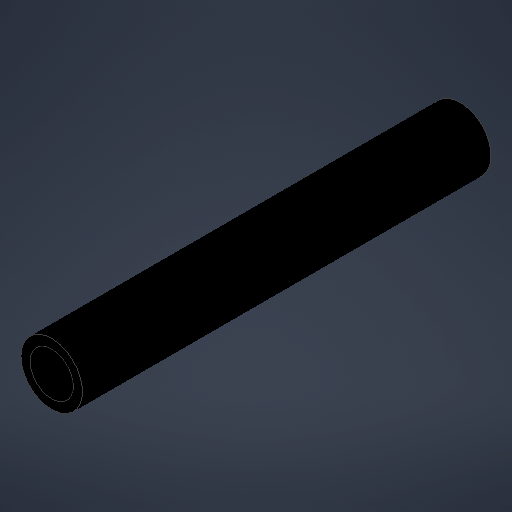
# Autodesk Inventor part: Dribbler Support
Saved by Autodesk Inventor 2026.1 (Build 301233020, 233B)
## iProperties
Created: 2025-12-15
Part Number: Dribbler Support
Material: Generic
Document SubType Name: Modeling
Designer: Bahaa
Density: 1 g/cm^3
Appearance: Default
Author: Bahaa
Autodesk Inventor part; units mm, degrees
ref_plane "YZ Plane" through (0, 0, 0) normal (1, 0, 0) x (0, 1, 0)
ref_plane "XZ Plane" through (0, 0, 0) normal (0, 1, 0) x (-1, 0, 0)
ref_plane "XY Plane" through (0, 0, 0) normal (0, 0, 1) x (1, 0, 0)
sketch "Sketch1" plane through (0, 0, 0) normal (0, 1, 0) x (-1, 0, 0)
  circle A0 centre (0, 0) radius 3
  dimension "d0" = 6
  constraints: 1 centre point, 1 coincident
  measures "d0" diameter of A0
extrude "Extrusion1" add sketch "Sketch1" along normal blind 39.8
hole "Hole1" at (0, 0, 0) direction (0, 1, 0) diameter 4.2 depth 6
sketch "Sketch2" plane through (0, 39.8, 0) normal (0, 1, 0) x (1, 0, 0)
  point P0 (0, 0)
hole "Hole2" at (0, 39.8, 0) direction (0, -1, 0) diameter 4.2 depth 6
body "Solid1"
